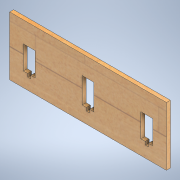
# Autodesk Inventor part: HolzServoHalter1
Saved by Autodesk Inventor 2020.3 (Build 243373010, 373A)
## iProperties
Created: 2020-12-09
Part Number: HolzServoHalter1
Material: Generisch
Document SubType Name: Modeling
Designer: Stefan
Density: 1 g/cm^3
Appearance: Ahorn - Galliano
Author: Stefan
Autodesk Inventor part; units mm, degrees
ref_plane "YZ Plane" through (0, 0, 0) normal (1, 0, 0) x (0, 1, 0)
ref_plane "XZ Plane" through (0, 0, 0) normal (0, 1, 0) x (-1, 0, 0)
ref_plane "XY Plane" through (0, 0, 0) normal (0, 0, 1) x (1, 0, 0)
sketch "Skizze1" plane through (0, 0, 0) normal (0, 0, 1) x (1, 0, 0)
  line L0 (0, 0) -> (400, 0)
  line L1 (400, 0) -> (400, -150)
  line L2 (400, -150) -> (0, -150)
  line L3 (0, -150) -> (0, 0)
  line L4 (35, -113) -> (35, -53)
  line L5 (35, -53) -> (65, -53)
  line L6 (65, -53) -> (65, -113)
  line L7 (185, -48) -> (215, -48)
  line L8 (215, -48) -> (215, -113)
  line L9 (185, -113) -> (185, -48)
  line L10 (335, -53) -> (365, -53)
  line L11 (365, -53) -> (365, -113)
  line L12 (335, -113) -> (335, -53)
  line L13 (204, -113) -> (204, -121)
  line L14 (204, -121) -> (196, -121)
  line L15 (196, -121) -> (196, -113)
  line L16 (215, -113) -> (204, -113)
  line L17 (196, -113) -> (185, -113)
  line L18 (54, -113) -> (54, -121)
  line L19 (54, -121) -> (46, -121)
  line L20 (46, -121) -> (46, -113)
  line L21 (65, -113) -> (54, -113)
  line L22 (46, -113) -> (35, -113)
  line L23 (354, -113) -> (354, -121)
  line L24 (354, -121) -> (346, -121)
  line L25 (346, -121) -> (346, -113)
  line L26 (365, -113) -> (354, -113)
  line L27 (346, -113) -> (335, -113)
  dimension "d0" = 400
  dimension "d1" = 150
  dimension "d2" = 65
  dimension "d3" = 30
  dimension "d4" = 30
  dimension "d5" = 60
  dimension "d6" = 30
  dimension "d7" = 60
  dimension "d8" = 35
  dimension "d12" = 35
  dimension "d13" = 185
  dimension "d16" = 8
  dimension "d17" = 8
  dimension "d18" = 11
  dimension "d19" = 8
  dimension "d20" = 8
  dimension "d21" = 11
  dimension "d22" = 8
  dimension "d23" = 8
  dimension "d24" = 11
  constraints: 56 end point, 14 parallel, 5 horizontal, 5 perpendicular, 1 coincident
  measures "d0" distance of L1.end L2.end
  measures "d1" distance of L0.end L1.end
  measures "d2" distance of L7.end L8.end
  measures "d3" distance of L7.start L7.end
  measures "d4" distance of L4.end L5.end
  measures "d5" distance of L5.end L6.end
  measures "d6" distance of L11.end L12.start
  measures "d7" distance of L10.end L11.end
  measures "d8" distance between parallel lines of L1 L11
  measures "d12" distance between parallel lines of L3 L4
  measures "d13" distance between parallel lines of L9 L3
  measures "d16" distance of L13.end L14.end
  measures "d17" distance of L13.start L13.end
  measures "d18" distance between parallel lines of L8 L13
  measures "d19" distance of L18.end L19.end
  measures "d20" distance of L18.start L18.end
  measures "d21" distance between parallel lines of L6 L18
  measures "d22" distance of L23.end L24.end
  measures "d23" distance of L23.start L23.end
  measures "d24" distance between parallel lines of L11 L23
extrude "Extrusion1" add sketch "Skizze1" along normal blind 10
